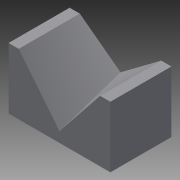
# Autodesk Inventor part: LoftCut
Saved by Autodesk Inventor 2015 (Build 190159000, 159)
## iProperties
Created: 2018-01-04
Part Number: LoftCut
Material: Generic
Document SubType Name: Modeling
Designer: Administrator
Density: 1 g/cm^3
Appearance: Default
Author: Administrator
Autodesk Inventor part; units mm, degrees
ref_plane "YZ Plane" through (0, 0, 0) normal (1, 0, 0) x (0, 1, 0)
ref_plane "XZ Plane" through (0, 0, 0) normal (0, 1, 0) x (-1, 0, 0)
ref_plane "XY Plane" through (0, 0, 0) normal (0, 0, 1) x (1, 0, 0)
sketch "Sketch1" plane through (0, 0, 0) normal (0, 0, 1) x (1, 0, 0)
  line L0 (0, 0) -> (63.5, 0)
  line L1 (63.5, 0) -> (63.5, 38.1)
  line L2 (63.5, 38.1) -> (0, 38.1)
  line L3 (0, 38.1) -> (0, 0)
  dimension "d0" = 38.1
  dimension "d1" = 63.5
  constraints: 8 end point, 2 parallel, 1 horizontal, 1 perpendicular
  measures "d0" distance of L2.end L0.start
  measures "d1" distance of L0.start L0.end
extrude "Extrusion1" add sketch "Sketch1" along normal blind 38.1
sketch "Sketch2" plane through (0, 0, 38.1) normal (0, 0, 1) x (1, 0, 0)
  line L0 (6.35, 38.1) -> (31.75, 6.35)
  line L1 (31.75, 6.35) -> (57.15, 38.1)
  line L2 (6.35, 38.1) -> (57.15, 38.1)
  point P0 (63.5, 38.1)
  point P1 (0, 38.1)
  dimension "d4" = 6.35
  dimension "d5" = 6.35
  constraints: 6 end point
  measures "d4" distance of L0.start point (0, 38.1)
  measures "d5" distance of point (63.5, 38.1) L1.end
sketch "Sketch3" plane through (0, 0, 0) normal (0, 0, -1) x (-1, 0, 0)
  line L0 (-57.15, 38.1) -> (-31.75, 19.05)
  line L1 (-31.75, 19.05) -> (-6.35, 38.1)
  line L2 (-57.15, 38.1) -> (-6.35, 38.1)
  line L3 (-63.5, 0) -> (-63.5, 38.1) projected
  line L4 (0, 38.1) -> (0, 0) projected
  line L5 (0, 0) -> (-63.5, 0) projected
  dimension "d8" = 6.35
  dimension "d9" = 6.35
  dimension "d10" = 19.05
  dimension "d11" = 31.75
  constraints: 6 end point
  measures "d8" distance from line of L3 L0.start
  measures "d9" distance from line of L4 L1.end
  measures "d10" distance from line of L5 L0.end
  measures "d11" distance from line of L3 L0.end
loft "Loft1" cut profiles "Sketch2", "Sketch3"
body "Solid1"
